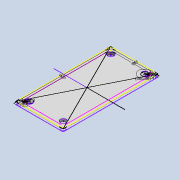
# Autodesk Inventor part: proper shit spodnji
Saved by Autodesk Inventor 2020 (Build 240168000, 168)
## iProperties
Created: 2020-08-03
Part Number: proper shit spodnji
Material: Generic
Document SubType Name: Modeling
Designer: borbu
Density: 1 g/cm^3
Appearance: Default
Author: borbu
Autodesk Inventor part; units mm, degrees
ref_plane "YZ Plane" through (0, 0, 0) normal (1, 0, 0) x (0, 1, 0)
ref_plane "XZ Plane" through (0, 0, 0) normal (0, 1, 0) x (-1, 0, 0)
ref_plane "XY Plane" through (0, 0, 0) normal (0, 0, 1) x (1, 0, 0)
sketch "Sketch1" plane through (0, 0, 0) normal (0, 1, 0) x (-1, 0, 0)
  line L0 (-18.75, 52.5) -> (26.25, 52.5)
  line L1 (26.25, 52.5) -> (26.25, -37.5)
  line L2 (26.25, -37.5) -> (-18.75, -37.5)
  line L3 (-18.75, -37.5) -> (-18.75, 52.5)
  line L4 (26.25, 52.5) -> (-18.75, -37.5) construction
  line L5 (-16.4706, 50) -> (23.5294, 50)
  line L6 (23.5294, 50) -> (23.5294, -35)
  line L7 (23.5294, -35) -> (-16.4706, -35)
  line L8 (-16.4706, -35) -> (-16.4706, 50)
  line L9 (23.5294, 50) -> (-16.4706, -35) construction
  line L10 (23.5294, 50) -> (21.0294, 50)
  line L11 (21.0294, 50) -> (21.0294, 47.5)
  line L12 (21.0294, 47.5) -> (23.5294, 47.5)
  line L13 (23.5294, 47.5) -> (23.5294, 50)
  arc A0 (23.5294, 47.5) -> (21.0294, 50) centre (21.0294, 47.5) ccw
  line L14 (26.25, 52.5) -> (22.75, 52.5)
  line L15 (22.75, 52.5) -> (22.75, 49)
  line L16 (22.75, 49) -> (26.25, 49)
  line L17 (26.25, 49) -> (26.25, 52.5)
  line L18 (23.5294, -35) -> (21.0294, -35)
  line L19 (21.0294, -35) -> (21.0294, -32.5)
  line L20 (21.0294, -32.5) -> (23.5294, -32.5)
  line L21 (23.5294, -32.5) -> (23.5294, -35)
  line L22 (-16.4706, -35) -> (-13.9706, -35)
  line L23 (-13.9706, -35) -> (-13.9706, -32.5)
  line L24 (-13.9706, -32.5) -> (-16.4706, -32.5)
  line L25 (-16.4706, -32.5) -> (-16.4706, -35)
  line L26 (-16.4706, 50) -> (-13.9706, 50)
  line L27 (-13.9706, 50) -> (-13.9706, 47.5)
  line L28 (-13.9706, 47.5) -> (-16.4706, 47.5)
  line L29 (-16.4706, 47.5) -> (-16.4706, 50)
  arc A1 (-13.9706, 50) -> (-16.4706, 47.5) centre (-13.9706, 47.5) ccw
  arc A2 (-16.4706, -32.5) -> (-13.9706, -35) centre (-13.9706, -32.5) ccw
  arc A3 (21.0294, -35) -> (23.5294, -32.5) centre (21.0294, -32.5) ccw
  arc A4 (26.25, 49) -> (22.75, 52.5) centre (22.75, 49) ccw
  line L30 (26.25, -37.5) -> (22.75, -37.5)
  line L31 (22.75, -37.5) -> (22.75, -34)
  line L32 (22.75, -34) -> (26.25, -34)
  line L33 (26.25, -34) -> (26.25, -37.5)
  line L34 (-18.75, -37.5) -> (-15.25, -37.5)
  line L35 (-15.25, -37.5) -> (-15.25, -34)
  line L36 (-15.25, -34) -> (-18.75, -34)
  line L37 (-18.75, -34) -> (-18.75, -37.5)
  line L38 (-18.75, 52.5) -> (-15.25, 52.5)
  line L39 (-15.25, 52.5) -> (-15.25, 49)
  line L40 (-15.25, 49) -> (-18.75, 49)
  line L41 (-18.75, 49) -> (-18.75, 52.5)
  arc A5 (-15.25, 52.5) -> (-18.75, 49) centre (-15.25, 49) ccw
  arc A6 (-18.75, -34) -> (-15.25, -37.5) centre (-15.25, -34) ccw
  arc A7 (22.75, -37.5) -> (26.25, -34) centre (22.75, -34) ccw
  point P0 (0, 0)
  point P1 (26.25, 49)
  point P2 (22.75, 52.5)
  point P3 (-18.75, -34)
  point P4 (-16.4706, -32.5)
  point P5 (-15.9706, -34)
  point P6 (-16.4706, -34)
  point P7 (23.5294, -32.5)
  dimension "d0" = 45
  dimension "d1" = 90
  dimension "d2" = 40
  dimension "d3" = 85
  dimension "d8" = 2.5
  dimension "d9" = 2.5
  constraints: 84 end point, 20 parallel, 16 point on circle, 10 horizontal, 10 perpendicular, 8 centre point, 8 coincident, 3 point on line
  measures "d0" distance of L1.end L2.end
  measures "d1" distance of L0.end L1.end
  measures "d2" distance of L6.end L7.end
  measures "d3" distance of L5.end L6.end
  measures "d8" distance of L12.end L11.end
  measures "d9" distance of L11.end L10.end
extrude "Extrusion3" add sketch "Sketch1" along normal blind 2.5 contours L0 L15 L5 L39 | L39 L5 L8 L40 A5 | L40 L8 L36 L3 | A4 L16 L6 L5 L15 | L39 A1 L40 L8 L5 | L5 A1 L39 | L36 L8 L7 L35 A6 | L40 A1 L8 | L15 A0 L5 | L5 L6 L16 A0 L15 | L1 L32 L6 L16 | L5 L11 L12 L6 L20 L19 L7 L23 L24 L8 L28 L27 | L27 L28 A1 L40 L39 | L39 L40 A1 | L36 A2 L35 L7 L8 | L35 L7 L31 L2 | A0 L15 L16 L12 L11 | A0 L16 L15 | A7 L31 L7 L6 L32 | L6 A0 L16 | L24 L23 A2 L35 L36 | L36 L35 A2 | L35 A2 L7 | L32 A3 L6 | L6 L7 L31 A3 L32 | L7 A3 L31 | A3 L32 L31 L19 L20 | A3 L31 L32
fillet "Fillet1" radius 3 8 edges at (-25.2249, 0, 51.4749) (-3.75, 0, 52.5) (17.7249, 0, 51.4749) (18.75, 0, 7.5) (17.7249, 0, -36.4749) (-3.75, 0, -37.5) (-25.2249, 0, -36.4749) (-26.25, 0, 7.5)
sketch "Sketch2" plane through (0, 2.5, 0) normal (0, 1, 0) x (1, 0, 0)
  arc A0 (16.4706, 32.5) -> (13.9706, 35) centre (13.9706, 32.5) ccw projected
  line L0 (13.9706, 35) -> (13.9706, 33.5)
  line L1 (16.4706, -47.5) -> (16.4706, 32.5) projected
  line L2 (16.4706, 32.5) -> (14.9706, 32.5)
  line L3 (14.9706, 32.5) -> (13.9706, 33.5)
  line L4 (14.4706, 33) -> (12.526, 31.0555)
  circle A1 centre (12.526, 31.0555) radius 2.75
  line L5 (-23.5294, 32.5) -> (-23.5294, -47.5) projected
  line L6 (-23.5294, -47.5) -> (-22.0294, -47.5)
  line L7 (-21.0294, -50) -> (13.9706, -50) projected
  line L8 (-21.0294, -50) -> (-21.0294, -48.5)
  line L9 (-21.0294, -48.5) -> (-22.0294, -47.5)
  line L10 (-21.5294, -48) -> (-19.5849, -46.0555)
  line L11 (-21.5294, -48) -> (-18.7794, -48) construction
  circle A2 centre (-19.5849, -46.0555) radius 2.75
  arc A3 (14.0518, 28.7675) -> (15.276, 31.0555) centre (12.526, 31.0555) ccw construction
  arc A4 (14.321, 28.3639) -> (15.7612, 31.0555) centre (12.526, 31.0555) ccw
  arc A5 (13.7826, 29.1712) -> (14.7909, 31.0555) centre (12.526, 31.0555) ccw
  arc A6 (13.7826, 29.1712) -> (14.321, 28.3639) centre (14.0518, 28.7675) ccw
  arc A7 (15.7612, 31.0555) -> (14.7909, 31.0555) centre (15.276, 31.0555) ccw
  arc A8 (10.7311, 33.747) -> (9.2909, 31.0555) centre (12.526, 31.0555) ccw
  arc A9 (9.2909, 31.0555) -> (10.2612, 31.0555) centre (9.776, 31.0555) ccw
  arc A10 (11.2694, 32.9398) -> (10.7311, 33.747) centre (11.0003, 33.3434) ccw
  arc A11 (11.2694, 32.9398) -> (10.2612, 31.0555) centre (12.526, 31.0555) ccw
  arc A12 (-17.79, -48.747) -> (-16.3497, -46.0555) centre (-19.5849, -46.0555) ccw
  arc A13 (-18.3283, -47.9398) -> (-17.32, -46.0555) centre (-19.5849, -46.0555) ccw
  arc A14 (-18.3283, -47.9398) -> (-17.79, -48.747) centre (-18.0591, -48.3434) ccw
  arc A15 (-16.3497, -46.0555) -> (-17.32, -46.0555) centre (-16.8349, -46.0555) ccw
  arc A16 (-21.3798, -43.3639) -> (-22.82, -46.0555) centre (-19.5849, -46.0555) ccw
  arc A17 (-22.82, -46.0555) -> (-21.8497, -46.0555) centre (-22.3349, -46.0555) ccw
  arc A18 (-20.8415, -44.1712) -> (-21.3798, -43.3639) centre (-21.1106, -43.7675) ccw
  arc A19 (-20.8415, -44.1712) -> (-21.8497, -46.0555) centre (-19.5849, -46.0555) ccw
  line L12 (-22.8137, -49.2843) -> (-20.2452, -46.7157) construction
  line L13 (-22.3894, -49.7085) -> (-19.8209, -47.14)
  line L14 (-20.6694, -46.2915) -> (-23.2379, -48.86)
  arc A20 (-23.2379, -48.86) -> (-22.3894, -49.7085) centre (-22.8137, -49.2843) ccw
  arc A21 (-19.8209, -47.14) -> (-20.6694, -46.2915) centre (-20.2452, -46.7157) ccw
  line L15 (12.9911, 31.5205) -> (15.9501, 34.4795) construction
  line L16 (13.4153, 31.0962) -> (16.3744, 34.0552)
  line L17 (15.5258, 34.9038) -> (12.5668, 31.9448)
  arc A22 (12.5668, 31.9448) -> (13.4153, 31.0962) centre (12.9911, 31.5205) ccw
  arc A23 (16.3744, 34.0552) -> (15.5258, 34.9038) centre (15.9501, 34.4795) ccw
  arc A24 (15.25, -52.5) -> (18.75, -49) centre (15.25, -49) ccw projected
  line L18 (15.25, -52.5) -> (18.75, -52.5)
  line L19 (18.75, -52.5) -> (18.75, -49)
  arc A25 (-22.75, 37.5) -> (-26.25, 34) centre (-22.75, 34) ccw projected
  line L20 (-26.25, 34) -> (-26.25, 37.5)
  line L21 (15.25, 37.5) -> (-22.75, 37.5) projected
  line L22 (-26.25, 37.5) -> (-22.75, 37.5)
  line L23 (-22.75, -52.5) -> (15.25, -52.5) projected
  line L24 (-22.75, -52.5) -> (-26.25, -52.5)
  line L25 (-26.25, 34) -> (-26.25, -49) projected
  line L26 (-26.25, -52.5) -> (-26.25, -49)
  line L27 (18.75, -49) -> (18.75, 34) projected
  line L28 (18.75, 37.5) -> (18.75, 34)
  line L29 (15.25, 37.5) -> (15.25, 34.542) projected
  line L30 (18.75, 37.5) -> (15.25, 37.5)
  line L31 (-26.25, -52.5) -> (18.75, 37.5)
  line L32 (18.75, -52.5) -> (-26.25, 37.5)
  line L33 (-3.75, -7.5) -> (32.3445, -7.5)
  line L34 (-35.1724, -7.5) -> (-3.75, -7.5)
  circle A26 centre (12.526, -46.0555) radius 2.75
  circle A27 centre (-19.5849, 31.0555) radius 2.75
  point P0 (0, 0)
  point P1 (14.848, 32.5289)
  point P2 (13.9995, 33.3774)
  point P3 (11.4261, 33.5759)
  point P4 (9.8188, 30.5722)
  point P5 (13.626, 28.535)
  point P6 (15.2333, 31.5387)
  point P7 (-21.9068, -47.5289)
  point P8 (-21.0583, -48.3774)
  point P9 (-18.4849, -48.5759)
  point P10 (-16.8777, -45.5722)
  point P11 (-20.6848, -43.535)
  point P12 (-22.2921, -46.5387)
  point P13 (15.2624, 34.6404)
  point P14 (16.111, 33.7918)
  point P15 (14.6612, -44.3223)
  point P16 (15.1936, -45.3873)
  dimension "d32" = 5.5
  dimension "d29" = 1.5
  dimension "d30" = 1.5
  dimension "d31" = 2.75
  dimension "d33" = 1.5
  dimension "d34" = 1.5
  dimension "d35" = 2.75
  dimension "d36" = 45
  dimension "d37" = 5.5
  dimension "d40" = 360
  dimension "d44" = 1.2
  dimension "d45" = 1.2
  constraints: 58 end point, 42 point on circle, 24 centre point, 19 tangent, 7 horizontal, 5 midpoint, 4 point on line, 4 vertical, 3 coincident, 3 perpendicular, 2 collinear, 2 parallel, 2 symmetric about line, 1 equal length, 29 other
  measures "d29" distance of L0.start L0.end
  measures "d30" distance of L1.end L2.end
  measures "d31" distance of L4.start L4.end
  measures "d33" distance of L5.end L6.end
  measures "d34" distance of L7.start L8.end
  measures "d35" distance of L10.start L10.end
  measures "d36" angle of L11 L10
  measures "d37" diameter of A2
  measures "d44" diameter of A21
  measures "d45" diameter of A23
extrude "Extrusion10" cut sketch "Sketch2" against normal blind 10 contours L32 A26 | A27 picked at (11.7147, -45.435)
sketch "Sketch4" plane through (0, 2.5, 0) normal (0, 1, 0) x (1, 0, 0)
  point P0 (0, 0)
body "Solid2"
